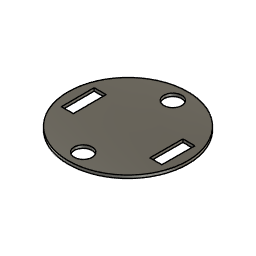
BAPS Robot (Autodesk Fusion 360 design; units mm, degrees)
Autodesk Fusion 360 part; units mm, degrees
sketch "No Need" plane through (0, 0, 0) normal (0, 0, 1) x (1, 0, 0)
  circle A0 centre (0, 0) radius 200
  line L0 (0, 0) -> (110, 0)
  line L1 (0, 0) -> (-110, 0)
  line L2 (-110, 0) -> (-110, 70)
  line L3 (110, 0) -> (110, 70)
  line L4 (110, 70) -> (-110, 70)
  line L5 (-110, 0) -> (-110, -70)
  line L6 (110, 0) -> (110, -70)
  line L7 (110, -70) -> (-110, -70)
  circle A1 centre (0, 0) radius 140
  dimension "d3" = 400
  dimension "d6" = 220
  dimension "d7" = 70
  dimension "d8" = 70
  dimension "d10" = 280
  constraint coincident A0.centre L0.start
  constraint horizontal L0
  constraint parallel L0 L1
  constraint perpendicular L1 L2
  constraint perpendicular L0 L3
  constraint perpendicular L2 L4
  constraint perpendicular L1 L5
  constraint perpendicular L0 L6
  measures "d3" diameter of A0
  measures "d6" distance of L0.end L1.end
  measures "d7" distance of L1.end L2.end
  measures "d8" distance of L1.end L5.end
  measures "d10" diameter of A1
sketch "Bottom Layer" plane through (0, 0, 0) normal (0, 0, 1) x (1, 0, 0)
  circle A0 centre (0, 0) radius 200
  line L0 (-168.2609, 0.0653) -> (-168.4591, 55.0649)
  line L1 (-168.2609, 0.0653) -> (-168.0627, -54.9343)
  line L2 (168.2609, 0.0653) -> (168.0627, -54.9343)
  line L3 (168.2609, 0.0653) -> (168.4591, 55.0649)
  line L4 (-168.4591, 55.0649) -> (-128.4594, 55.2091)
  line L5 (-128.4594, 55.2091) -> (-128.063, -54.7902)
  line L6 (-128.063, -54.7902) -> (-168.0627, -54.9343)
  line L7 (168.4591, 55.0649) -> (128.4594, 55.2091)
  line L8 (128.4594, 55.2091) -> (128.063, -54.7902)
  line L9 (128.063, -54.7902) -> (168.0627, -54.9343)
  circle A1 centre (0, 150) radius 30
  line L10 (0, 180) -> (0, 200)
  circle A2 centre (0, -150) radius 30
  line L11 (0, -180) -> (0, -200)
  dimension "d43" = 400
  dimension "d45" = 55
  dimension "d46" = 55
  dimension "d48" = 55
  dimension "d49" = 55
  dimension "d50" = 110
  dimension "d51" = 110
  dimension "d52" = 40
  dimension "d53" = 40
  dimension "d54" = 40
  dimension "d55" = 40
  dimension "d57" = 60
  dimension "d58" = 20
  dimension "d60" = 60
  dimension "d61" = 20
  constraint perpendicular L0 L4
  constraint perpendicular L1 L6
  constraint perpendicular L3 L7
  constraint perpendicular L2 L9
  constraint coincident A0 L10.end
  constraint coincident A1 L10.start
  constraint coincident A2 L11.start
  constraint coincident A0 L11.end
  constraint vertical L11
  measures "d43" diameter of A0
  measures "d45" distance of L0.start L0.end
  measures "d46" distance of L0.start L1.end
  measures "d48" distance of L2.start L2.end
  measures "d49" distance of L2.start L3.end
  measures "d50" distance of L4.end L5.end
  measures "d51" distance of L7.end L8.end
  measures "d52" distance of L3.end L7.end
  measures "d53" distance of L0.end L4.end
  measures "d54" distance of L1.end L5.end
  measures "d55" distance of L2.end L8.end
  measures "d57" diameter of A1
  measures "d58" distance of L10.end L10.start
  measures "d60" diameter of A2
  measures "d61" distance of L11.start L11.end
extrude "Extrude1" add sketch "Bottom Layer" along normal blind 10 makes body 1
extrude "Extrude2" add sketch "No Need" along normal blind 10 separate body contours A0 | L0 L1 L2 L3 L4 | L0 L1 L5 L6 L7 | A1 makes body 2
sketch "Top" plane through (0, 0, 0) normal (0, 0, 1) x (1, 0, 0)
  circle A0 centre (0, 0) radius 200
  dimension "d66" = 400
  constraint coincident A0.centre origin
  measures "d66" diameter of A0
extrude "Extrude3" [rolled back] along distance 10 taper angle 0
hidden bodies 2
named bodies: "Bottom", "Top"
